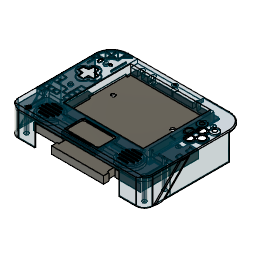
dsCase (Autodesk Fusion 360 design; units mm, degrees)
Autodesk Fusion 360 part; units mm, degrees
(part 1 of 7)
sketch "ds_pcb" plane through (0, 0, 0) normal (0, 0, 1) x (1, 0, 0)
  line L0 (0, 0) -> (0, 63.54)
  line L1 (125.8, 68.8) -> (125.8, 0)
  line L2 (0, 0) -> (0, 63.54)
  line L3 (0, 63.54) -> (24.68, 63.54)
  line L4 (24.68, 63.54) -> (24.68, 68.8)
  line L5 (24.68, 68.8) -> (88.18, 68.8)
  line L6 (24.68, 68.8) -> (88.18, 68.8)
  line L7 (88.18, 68.8) -> (24.68, 68.8)
  line L8 (103.34, 62.2) -> (113.8, 62.2)
  line L9 (125.8, 68.8) -> (115, 68.8)
  line L10 (125.8, 68.8) -> (113.8, 68.8)
  line L11 (113.8, 68.8) -> (113.8, 62.2)
  line L12 (125.8, 68.8) -> (113.8, 68.8)
  line L13 (113.8, 68.8) -> (125.8, 68.8)
  line L14 (88.3, 68.8) -> (88.18, 68.8)
  line L15 (94.8, 68.8) -> (102.3, 68.8)
  line L16 (102.3, 68.8) -> (102.3, 62.2)
  line L17 (102.3, 62.2) -> (103.34, 62.2)
  line L18 (88.3, 68.8) -> (88.3, 63)
  line L19 (94.8, 68.8) -> (94.8, 63)
  line L20 (94.8, 63) -> (88.3, 63)
  line L21 (28.46, 68.8) -> (28.46, 67.3) construction
  line L22 (28.46, 67.3) -> (28.46, 65.3) construction
  circle A0 centre (28.46, 65.3) radius 2
  line L23 (28.46, 65.3) -> (24.68, 65.3) construction
  line L24 (125.8, 68.8) -> (113.8, 68.8)
  line L25 (102.3, 68.8) -> (94.8, 68.8)
  line L26 (98.55, 68.8) -> (98.55, 67.4) construction
  line L27 (98.55, 67.4) -> (98.55, 65.4) construction
  circle A1 centre (98.55, 65.4) radius 2
  line L28 (0, 0) -> (0, 3.5)
  line L29 (0, 3.5) -> (3.5, 3.5) construction
  line L30 (3.5, 3.5) -> (1.5, 3.5) construction
  circle A2 centre (3.5, 3.5) radius 2
  line L31 (125.8, 0) -> (125.8, 3.5)
  line L32 (125.8, 3.5) -> (122.3, 3.5) construction
  line L33 (122.3, 3.5) -> (124.3, 3.5) construction
  circle A3 centre (122.3, 3.5) radius 2
  line L34 (0, 0) -> (34.7, 0)
  line L35 (125.8, 0) -> (96, 0)
  line L36 (37, 10.8) -> (34.7, 10.8)
  line L37 (34.7, 10.8) -> (34.7, 0)
  line L38 (93.7, 10.8) -> (96, 10.8)
  line L39 (96, 10.8) -> (96, 0)
  line L40 (0, 0) -> (34.7, 0)
  line L41 (96, 0) -> (125.8, 0)
  line L42 (72.4833, -13.7) -> (34.7, -13.7)
  line L43 (34.7, -13.7) -> (34.7, -7.2)
  line L44 (72.4833, -13.7) -> (96, -13.7)
  line L45 (96, -13.7) -> (96, -7.2)
  line L46 (96, 10.8) -> (93.7, 10.8)
  line L47 (34.7, 10.8) -> (37, 10.8)
  line L48 (34.7, -13.7) -> (34.7, -7.2)
  line L49 (34.7, -7.2) -> (37, -7.2)
  line L50 (37, -7.2) -> (37, 10.8)
  line L51 (96, -13.7) -> (96, -7.2)
  line L52 (96, -7.2) -> (93.7, -7.2)
  line L53 (93.7, -7.2) -> (93.7, 10.8)
  dimension "d1" = 125.8
  dimension "d3" = 63.54
  dimension "d4" = 101.12
  dimension "d5" = 63.5
  dimension "d11" = 12
  dimension "d14" = 7.5
  dimension "d15" = 31
  dimension "d16" = 6.5
  dimension "d17" = 5.8
  dimension "d20" = 1.5
  dimension "d21" = 2
  dimension "d22" = 4
  dimension "d23" = 1.4
  dimension "d24" = 2
  dimension "d25" = 3.5
  dimension "d26" = 3.5
  dimension "d27" = 2
  dimension "d28" = 3.5
  dimension "d29" = 3.5
  dimension "d30" = 2
  dimension "d31" = 34.7
  dimension "d32" = 29.8
  dimension "d35" = 2.3
  dimension "d36" = 2.3
  dimension "d37" = 6.5
  dimension "d38" = 6.5
  constraint coincident L0.start L2.start
  constraint horizontal L40
  constraint perpendicular L0 L40
  constraint perpendicular L0 L6
  constraint perpendicular L1 L40
  constraint perpendicular L2 L40
  constraint perpendicular L1 L12
  constraint perpendicular L0 L3
  constraint perpendicular L3 L4
  constraint perpendicular L4 L5
  constraint collinear L7 L12
  constraint perpendicular L1 L9
  constraint perpendicular L1 L10
  constraint perpendicular L8 L11
  constraint perpendicular L8 L16
  constraint perpendicular L1 L24
  constraint perpendicular L14 L18
  constraint perpendicular L15 L19
  constraint perpendicular L18 L20
  constraint coincident L7 L21.start
  constraint perpendicular L7 L21
  constraint perpendicular L7 L22
  constraint coincident L22.end A0.centre
  constraint coincident L4 L23.end
  constraint perpendicular L4 L23
  constraint collinear L24 L25
  constraint midpoint L15 L26.start
  constraint perpendicular L15 L26
  constraint parallel L26 L27
  constraint coincident L27.end A1.centre
  constraint coincident L26.end A1
  constraint perpendicular L28 L40
  constraint perpendicular L28 L29
  constraint parallel L29 L30
  constraint coincident L29.end L30.start
  constraint coincident L30.end A2
  constraint perpendicular L31 L40
  constraint perpendicular L31 L32
  constraint parallel L32 L33
  constraint coincident L32.end L33.start
  constraint coincident L33.end A3
  constraint perpendicular L28 L34
  constraint perpendicular L1 L35
  constraint perpendicular L34 L37
  constraint perpendicular L39 L40
  constraint collinear L40 L41
  constraint perpendicular L37 L42
  constraint perpendicular L34 L43
  constraint perpendicular L39 L44
  constraint perpendicular L41 L45
  constraint perpendicular L39 L46
  constraint perpendicular L37 L47
  constraint perpendicular L42 L48
  constraint perpendicular L43 L49
  constraint perpendicular L47 L50
  constraint perpendicular L44 L51
  constraint perpendicular L45 L52
  constraint perpendicular L38 L53
  measures "d1" distance of L0.start L1.end
  measures "d3" distance of L0.start L0.end
  measures "d4" distance of L1.start L4.end
  measures "d5" distance of L4.end L5.end
  measures "d11" distance of L1.start L10.end
  measures "d14" distance of L15.start L15.end
  measures "d15" distance of L1.start L15.start
  measures "d16" distance of L15.start L14.start
  measures "d17" distance of L14.start L18.end
  measures "d20" distance of L21.start L21.end
  measures "d21" distance of L21.end L22.end
  measures "d22" diameter of A0
  measures "d23" distance of L26.start L26.end
  measures "d24" distance of L26.end L27.end
  measures "d25" distance of L0.start L28.end
  measures "d26" distance of L28.end L29.end
  measures "d27" distance of L29.end L30.end
  measures "d28" distance of L1.end L31.end
  measures "d29" distance of L31.end L32.end
  measures "d30" distance of L32.end L33.end
  measures "d31" distance of L0.start L34.end
  measures "d32" distance of L1.end L35.end
  measures "d35" distance of L38.end L38.start
  measures "d36" distance of L36.end L36.start
  measures "d37" distance of L42.end L43.end
  measures "d38" distance of L44.end L45.end
sketch "dsi_screen" plane through (0, 0, 0) normal (0, 0, 1) x (1, 0, 0)
  line L0 (0, 0) -> (0, 79.2)
  line L1 (0, 0) -> (93.9, 0)
  line L2 (0, 79.2) -> (93.9, 79.2)
  line L3 (93.9, 79.2) -> (93.9, 0)
  dimension "d39" = 79.2
  dimension "d40" = 93.9
  constraint coincident L0.start L1.start
  constraint vertical L0
  constraint perpendicular L0 L1
  constraint perpendicular L0 L2
  constraint perpendicular L1 L3
  measures "d39" distance of L0.start L0.end
  measures "d40" distance of L0.start L1.end
sketch "buttons" plane through (0, 0, 0) normal (0, 0, 1) x (1, 0, 0)
  line L0 (0, 0) -> (7.5, 0) construction
  line L1 (3.75, 0) -> (3.75, 3.75) construction
  line L2 (3.75, 0) -> (3.75, -3.75) construction
  line L3 (7.5, 0) -> (11.25, 0) construction
  line L4 (3.75, 3.75) -> (3.75, 7.5) construction
  line L5 (0, 0) -> (-3.75, 0) construction
  line L6 (3.75, -3.75) -> (3.75, -7.5) construction
  circle A0 centre (11.25, 0) radius 3.75
  circle A1 centre (3.75, 7.5) radius 3.75
  circle A2 centre (3.75, -7.5) radius 3.75
  circle A3 centre (-3.75, 0) radius 3.75
  line L7 (15, 0) -> (20, 0) construction
  line L8 (-7.5, 0) -> (-12.5, 0) construction
  line L9 (3.75, 11.25) -> (3.75, 16.25) construction
  line L10 (3.75, -11.25) -> (3.75, -16.25) construction
  line L11 (-12.5, 0) -> (-12.5, -16.25)
  line L12 (-12.5, -16.25) -> (3.75, -16.25)
  line L13 (3.75, -16.25) -> (20, -16.25)
  line L14 (20, -16.25) -> (20, 0)
  line L15 (20, 0) -> (20, 16.25)
  line L16 (20, 16.25) -> (3.75, 16.25)
  line L17 (3.75, 16.25) -> (-12.5, 16.25)
  line L18 (-12.5, 16.25) -> (-12.5, 0)
  line L19 (-12.5, 16.25) -> (-12.5, 26.25)
  line L20 (20, 16.25) -> (20, 26.25)
  line L21 (-12.5, 26.25) -> (20, 26.25)
  dimension "d41" = 7.5
  dimension "d42" = 3.75
  dimension "d43" = 3.75
  dimension "d44" = 3.75
  dimension "d45" = 3.75
  dimension "d46" = 3.75
  dimension "d47" = 3.75
  dimension "d48" = 5
  dimension "d49" = 5
  dimension "d50" = 5
  dimension "d51" = 5
  dimension "d93" = 10
  dimension "d94" = 10
  constraint coincident L0.start L5.start
  constraint horizontal L0
  constraint midpoint L0 L1.start
  constraint perpendicular L0 L1
  constraint perpendicular L0 L2
  constraint perpendicular L1 L3
  constraint parallel L1 L4
  constraint parallel L0 L5
  constraint parallel L2 L6
  constraint coincident L3.end A0.centre
  constraint coincident L0.end A0
  constraint coincident L4.end A1.centre
  constraint coincident L1.end A1
  constraint coincident L6.end A2.centre
  constraint coincident L2.end A2
  constraint coincident L5.end A3.centre
  constraint coincident L0.start A3
  constraint coincident A0 L7.start
  constraint horizontal L7
  constraint coincident A3 L8.start
  constraint parallel L7 L8
  constraint coincident A1 L9.start
  constraint parallel L4 L9
  constraint coincident A2 L10.start
  constraint perpendicular L5 L10
  constraint perpendicular L8 L11
  constraint perpendicular L10 L12
  constraint perpendicular L10 L13
  constraint perpendicular L7 L14
  constraint perpendicular L7 L15
  constraint perpendicular L9 L16
  constraint perpendicular L9 L17
  constraint perpendicular L8 L18
  constraint perpendicular L17 L19
  constraint perpendicular L16 L20
  measures "d41" distance of L0.start L0.end
  measures "d42" distance of L1.start L1.end
  measures "d43" distance of L1.start L2.end
  measures "d44" distance of L0.end L3.end
  measures "d45" distance of L1.end L4.end
  measures "d46" distance of L0.start L5.end
  measures "d47" distance of L2.end L6.end
  measures "d48" distance of L7.start L7.end
  measures "d49" distance of L8.start L8.end
  measures "d50" distance of L9.start L9.end
  measures "d51" distance of L10.start L10.end
  measures "d93" distance of L17.end L19.end
  measures "d94" distance of L15.end L20.end
sketch "cross" plane through (0, 0, 0) normal (0, 0, 1) x (1, 0, 0)
  line L0 (9.25, -9.25) -> (9.25, -16.25) construction
  line L1 (18.5, 0) -> (25.5, 0) construction
  line L2 (0, 0) -> (-7, 0) construction
  line L3 (0, 0) -> (0, 3.25)
  line L4 (0, 3.25) -> (0, -3.25)
  line L5 (18.5, 0) -> (18.5, 3.25)
  line L6 (18.5, 0) -> (18.5, -3.25)
  line L7 (9.25, 9.25) -> (12.5, 9.25)
  line L8 (9.25, 9.25) -> (6, 9.25)
  line L9 (9.25, -9.25) -> (12.5, -9.25)
  line L10 (9.25, -9.25) -> (6, -9.25)
  line L11 (9.25, 9.25) -> (9.25, 16.25) construction
  line L12 (0, 3.25) -> (6, 3.25)
  line L13 (12.5, 3.25) -> (18.5, 3.25)
  line L14 (6, 9.25) -> (6, 3.25)
  line L15 (6, -3.25) -> (6, -9.25)
  line L16 (12.5, 9.25) -> (12.5, 3.25)
  line L17 (12.5, -3.25) -> (12.5, -9.25)
  line L18 (0, -3.25) -> (6, -3.25)
  line L19 (12.5, -3.25) -> (18.5, -3.25)
  line L20 (9.25, 16.25) -> (-7, 16.25)
  line L21 (-7, 16.25) -> (-7, 0)
  line L22 (-7, 0) -> (-7, -16.25)
  line L23 (-7, -16.25) -> (9.25, -16.25)
  line L24 (9.25, -16.25) -> (25.5, -16.25)
  line L25 (25.5, -16.25) -> (25.5, 0)
  line L26 (25.5, 0) -> (25.5, 16.25)
  line L27 (25.5, 16.25) -> (9.25, 16.25)
  dimension "d52" = 18.5
  dimension "d59" = 3.25
  dimension "d60" = 6.5
  dimension "d61" = 3.25
  dimension "d62" = 3.25
  dimension "d63" = 3.25
  dimension "d64" = 3.25
  dimension "d65" = 3.25
  dimension "d66" = 3.25
  constraint coincident L2.start L3.start
  constraint perpendicular L2 L3
  constraint parallel L3 L4
  constraint perpendicular L0 L9
  constraint collinear L12 L13
  constraint collinear L14 L15
  constraint coincident L3 L2.start
  constraint collinear L16 L17
  constraint coincident L17.start L18
  constraint collinear L18 L19
  constraint perpendicular L11 L20
  constraint perpendicular L2 L21
  constraint perpendicular L2 L22
  constraint perpendicular L0 L23
  constraint perpendicular L0 L24
  constraint perpendicular L1 L25
  constraint perpendicular L20 L26
  constraint perpendicular L11 L27
  measures "d52" distance of L2.start L1.start
  measures "d59" distance of L2.start L3.end
  measures "d60" distance of L3.end L4.end
  measures "d61" distance of L1.start L5.end
  measures "d62" distance of L1.start L6.end
  measures "d63" distance of L7.start L7.end
  measures "d64" distance of L7.start L8.end
  measures "d65" distance of L0.start L9.end
  measures "d66" distance of L0.start L10.end
extrude "Extrude1" add sketch "dsi_screen" along normal blind 5.6 makes body 1
extrude "Extrude2" add sketch "ds_pcb" against normal blind 0.7 separate body makes body 2
move_body "Move1" bodies 1 to x (1, 0, 0) y (0, 1, 0) z (0, 0, 1) at (0, 0, 10)
extrude "Extrude3" add sketch "cross" along normal blind 2.5 separate body makes body 3
move_body "Move2" bodies 3 to x (1, 0, 0) y (0, 1, 0) z (0, 0, 1) at (-30, 60, 12)
sketch "Sketch5" plane through (0, 0, 15.6) normal (0, 0, 1) x (-1, 0, 0)
  line L0 (0, 0) -> (-93.9, 0)
  line L1 (-93.9, 0) -> (-93.9, -79.2)
  line L2 (-93.9, -79.2) -> (0, -79.2)
  line L3 (0, -79.2) -> (0, 0)
  line L4 (0, -79.2) -> (0, -57.7) construction
  line L5 (0, -57.7) -> (-93.9, -57.7) construction
  dimension "d75" = 21.5
  constraint coincident L2.end L3.start
  constraint perpendicular L2 L4
  constraint coincident L1 L5.end
  constraint perpendicular L1 L5
  measures "d75" distance of L2.end L4.end
move_body "Move4" bodies 3 to x (1, 0, 0) y (0, 1, 0) z (0, 0, 1) at (-2, 0, 0)
move_body "Move5" bodies 3 to x (1, 0, 0) y (0, 1, 0) z (0, 0, 1) at (6.5, -18.55, 1.1)
extrude "Extrude5" add sketch "buttons" along normal blind 2.5 separate body makes body 4
move_body "Move7" bodies 4 to x (1, 0, 0) y (0, 1, 0) z (0, 0, 1) at (106.4, 31.45, 13.1)
move_body "Move8" bodies 1 to x (1, 0, 0) y (0, 1, 0) z (0, 0, 1) at (0, -4.1, 0)
move_body "Move9" bodies 4 to x (1, 0, 0) y (0, 1, 0) z (0, 0, 1) at (0, 10, 0)
sketch "Sketch14" plane through (0, 0, 15.6) normal (0, 0, 1) x (-1, 0, 0)
  circle A0 centre (-102.65, -41.45) radius 3.75
  circle A1 centre (-110.15, -33.95) radius 3.75
  circle A2 centre (-117.65, -41.45) radius 3.75
  circle A3 centre (-110.15, -48.95) radius 3.75
  line L0 (-93.9, -67.7) -> (-93.9, -25.2)
  line L1 (-93.9, -25.2) -> (-126.4, -25.2)
  line L2 (-126.4, -25.2) -> (-126.4, -67.7)
  line L3 (-126.4, -67.7) -> (-93.9, -67.7)
  line L4 (-110.15, -48.95) -> (-117.65, -41.45) construction
  line L5 (-117.65, -41.45) -> (-110.15, -41.45) construction
  line L6 (-110.15, -41.45) -> (-110.15, -48.95) construction
  line L7 (-110.15, -48.95) -> (-102.6547, -56.4453) construction
  line L8 (-110.15, -48.95) -> (-117.6453, -56.4453) construction
  circle A4 centre (-102.6547, -56.4453) radius 2.35
  circle A5 centre (-117.6453, -56.4453) radius 2.35
  dimension "d96" = 10.6
  dimension "d97" = 10.6
  dimension "d98" = 4.7
  dimension "d99" = 4.7
  constraint coincident A3.centre L4.start
  constraint coincident A2.centre L4.end
  constraint horizontal L5
  constraint perpendicular L5 L6
  constraint parallel L4 L7
  constraint perpendicular L4 L8
  constraint coincident L7.end A4.centre
  constraint coincident L8.end A5.centre
  measures "d96" distance of A3.centre L7.end
  measures "d97" distance of A3.centre L8.end
  measures "d98" diameter of A4
  measures "d99" diameter of A5
extrude "Extrude7" cut sketch "Sketch14" against normal blind 3 contours A4 | A5 bodies 4
sketch "Sketch15" plane through (0, 0, 15.6) normal (0, 0, 1) x (-1, 0, 0)
  line L0 (0, 4.1) -> (-93.9, 4.1)
  line L1 (-93.9, 4.1) -> (-93.9, -75.1)
  line L2 (-93.9, -75.1) -> (0, -75.1)
  line L3 (0, -75.1) -> (0, 4.1)
  line L4 (-46.95, -75.1) -> (-46.95, -85.1)
  line L5 (-46.95, -85.1) -> (32.5, -85.1)
  line L6 (32.5, -85.1) -> (32.5, -57.7)
  line L7 (32.5, -57.7) -> (0, -57.7)
  line L8 (0, -75.1) -> (0, -57.7)
  line L9 (0, -75.1) -> (-93.9, -75.1)
  line L10 (-93.9, -75.1) -> (-93.9, -67.7)
  line L11 (-93.9, -67.7) -> (-126.4, -67.7)
  line L12 (-126.4, -67.7) -> (-126.4, -85.1)
  line L13 (-126.4, -85.1) -> (-46.95, -85.1)
  point P0 (32.5, -57.7)
  point P1 (0, -57.7)
  point P2 (0, -57.7)
  point P3 (-93.9, -67.7)
  point P4 (-93.9, -67.7)
  point P5 (-126.4, -67.7)
  dimension "d102" = 10
  constraint midpoint L2 L4.start
  constraint perpendicular L2 L4
  constraint perpendicular L4 L5
  constraint coincident P0 L6.end
  constraint perpendicular L5 L6
  constraint coincident P2 P1
  constraint coincident L2.end L3.start
  constraint coincident L1.end L2.start
  constraint coincident P4 P3
  constraint coincident P5 L11.end
  constraint perpendicular L5 L12
  constraint perpendicular L4 L13
  measures "d102" distance of L4.start L4.end
extrude "Extrude8" add sketch "Sketch15" against normal blind 2.5 separate body contours L2 L3 L4 L5 L6 L7 L8 L9 | L1 L2 L4 L9 L10 L11 L12 L13 makes body 5
sketch "Sketch16" plane through (0, 0, 15.6) normal (0, 0, 1) x (-1, 0, 0)
  line L0 (0, -75.1) -> (-93.9, -75.1)
  line L1 (-93.9, -75.1) -> (-93.9, -67.7)
  line L2 (-93.9, -67.7) -> (-126.4, -67.7)
  line L3 (-126.4, -67.7) -> (-126.4, -85.1)
  line L4 (-126.4, -85.1) -> (32.5, -85.1)
  line L5 (32.5, -85.1) -> (32.5, -57.7)
  line L6 (32.5, -57.7) -> (0, -57.7)
  line L7 (0, -57.7) -> (0, -75.1)
  line L8 (-126.4, -85.1) -> (-106.4, -85.1)
  line L9 (-106.4, -85.1) -> (-106.4, -65.1)
  line L10 (-126.4, -85.1) -> (-126.4, -65.1)
  arc A0 (-126.4, -65.1) -> (-106.4, -85.1) centre (-106.4, -65.1) ccw
  line L11 (-46.95, -75.1) -> (-46.95, -92.0234) construction
  arc A1 (12.5, -85.1) -> (32.5, -65.1) centre (12.5, -65.1) ccw
  line L12 (32.5, -85.1) -> (32.5, -65.1)
  line L13 (32.5, -85.1) -> (12.5, -85.1)
  dimension "d105" = 20
  dimension "d106" = 20
  constraint coincident L3.end L4.start
  constraint perpendicular L3 L8
  constraint perpendicular L2 L9
  constraint coincident L9.end A0.centre
  constraint tangent L10 A0
  constraint midpoint L0 L11.start
  constraint perpendicular L4 L11
  constraint symmetric L3.end L11 L4.end
  constraint symmetric L8.end L11 A1.start
  constraint symmetric L10.end L11 A1.end
  constraint symmetric A0 L11 A1
  measures "d105" distance of L3.end L8.end
  measures "d106" distance of L8.end L9.end
extrude "Extrude9" cut sketch "Sketch16" against normal blind 2.5 contours L4 L5 A1 L12 L13 | L2 L3 L4 L8 L10 A0 | L2 L10 A0 bodies 4 5
sketch "Controls" plane through (0, 0, 15.6) normal (0, 0, 1) x (-1, 0, 0)
  line L0 (0, 4.1) -> (-93.9, 4.1)
  line L1 (-93.9, 4.1) -> (-93.9, -75.1)
  line L2 (-93.9, -75.1) -> (0, -75.1)
  line L3 (0, -75.1) -> (0, 4.1)
  line L4 (-93.9, 4.1) -> (0, 4.1)
  line L5 (0, 4.1) -> (0, -75.1)
  line L6 (0, -75.1) -> (-93.9, -75.1)
  line L7 (-93.9, -75.1) -> (-93.9, 4.1)
  line L8 (0, -25.2) -> (32.5, -25.2)
  line L9 (32.5, -25.2) -> (32.5, -65.1)
  arc A0 (12.5, -85.1) -> (32.5, -65.1) centre (12.5, -65.1) ccw
  line L10 (12.5, -85.1) -> (-106.4, -85.1)
  line L11 (-93.9, -25.2) -> (-126.4, -25.2)
  line L12 (-126.4, -25.2) -> (-93.9, -25.2)
  arc A1 (12.5, -85.1) -> (32.5, -65.1) centre (12.5, -65.1) ccw
  line L13 (-126.4, -25.2) -> (-126.4, -65.1)
  arc A2 (-126.4, -65.1) -> (-106.4, -85.1) centre (-106.4, -65.1) ccw
  line L14 (19.5, -44.7) -> (19.5, -50.7)
  line L15 (19.5, -50.7) -> (19.5, -44.7)
  line L16 (19.5, -44.7) -> (25.5, -44.7)
  line L17 (25.5, -44.7) -> (25.5, -38.2)
  line L18 (25.5, -38.2) -> (19.5, -38.2)
  line L19 (19.5, -38.2) -> (19.5, -32.2)
  line L20 (19.5, -32.2) -> (13, -32.2)
  line L21 (13, -32.2) -> (13, -38.2)
  line L22 (13, -38.2) -> (7, -38.2)
  line L23 (7, -38.2) -> (7, -44.7)
  line L24 (7, -44.7) -> (13, -44.7)
  line L25 (13, -44.7) -> (13, -50.7)
  line L26 (13, -50.7) -> (19.5, -50.7)
  circle A3 centre (-117.65, -41.45) radius 3.75
  circle A4 centre (-110.15, -48.95) radius 3.75
  circle A5 centre (-110.15, -33.95) radius 3.75
  circle A6 centre (-117.65, -41.45) radius 3.75
  circle A7 centre (-110.15, -48.95) radius 3.75
  circle A8 centre (-110.15, -33.95) radius 3.75
  circle A9 centre (-102.65, -41.45) radius 3.75
  circle A10 centre (-102.6547, -56.4453) radius 2.35
  circle A11 centre (-102.6547, -56.4453) radius 2.35
  circle A12 centre (-117.6453, -56.4453) radius 2.35
  circle A13 centre (-102.6547, -56.4453) radius 2.35
  circle A14 centre (-117.6453, -56.4453) radius 2.35
  line L27 (-110.15, -33.95) -> (-110.15, -40) construction
  line L28 (-110.15, -33.95) -> (-110.15, -37.7) construction
  line L29 (-110.15, -37.7) -> (-110.15, 35.3) construction
  line L30 (-126.4, -25.2) -> (-126.4, 25.3)
  line L31 (32.5, -25.2) -> (32.5, 25.3)
  line L32 (-110.15, 35.3) -> (-116.4, 35.3)
  line L33 (-110.15, 35.3) -> (22.5, 35.3)
  line L34 (0, 4.1) -> (0, 35.3) construction
  circle A15 centre (0, 19.7) radius 11.5
  line L35 (-93.9, 4.1) -> (-93.9, 35.3) construction
  circle A16 centre (-93.9, 19.7) radius 11.5
  line L36 (-116.4, 35.3) -> (-116.4, 25.3) construction
  arc A17 (-116.4, 35.3) -> (-126.4, 25.3) centre (-116.4, 25.3) ccw
  line L37 (22.5, 35.3) -> (22.5, 25.3) construction
  arc A18 (32.5, 25.3) -> (22.5, 35.3) centre (22.5, 25.3) ccw
  point P0 (0, -25.2)
  point P1 (32.5, -25.2)
  point P2 (-126.2303, -67.7)
  point P3 (-126.4, -25.2)
  point P4 (-126.4, -25.2)
  point P5 (-93.9, -25.2)
  point P6 (19.5, -50.7)
  point P7 (19.5, -44.7)
  point P8 (19.5, -44.7)
  point P9 (25.5, -44.7)
  point P10 (25.5, -38.2)
  point P11 (19.5, -38.2)
  point P12 (19.5, -32.2)
  point P13 (13, -32.2)
  point P14 (13, -38.2)
  point P15 (7, -38.2)
  point P16 (7, -44.7)
  point P17 (13, -44.7)
  point P18 (13, -50.7)
  point P19 (-98.9, -41.45)
  point P20 (-119.9953, -56.4453)
  dimension "d127" = 73
  dimension "d128" = 23
  dimension "d129" = 23
  dimension "d131" = 10
  dimension "d133" = 10
  constraint coincident L0.end L1.start
  constraint coincident L0.start L3.end
  constraint coincident L2.end L3.start
  constraint coincident L1.end L2.start
  constraint coincident P0 L8.start
  constraint coincident P1 L8.end
  constraint coincident L9.end A0.end
  constraint coincident A0.start L10.start
  constraint coincident L10.end A2.end
  constraint coincident P4 P3
  constraint coincident P5 L11.start
  constraint concentric A0 A1
  constraint coincident L13.end A2.start
  constraint coincident L13.end A2
  constraint coincident P6 L14.end
  constraint coincident P8 P7
  constraint coincident P9 L16.end
  constraint coincident P10 L17.end
  constraint coincident P11 L18.end
  constraint coincident P12 L19.end
  constraint coincident P13 L20.end
  constraint coincident P14 L21.end
  constraint coincident P15 L22.end
  constraint coincident P16 L23.end
  constraint coincident P17 L24.end
  constraint coincident P18 L25.end
  constraint concentric A3 A6
  constraint concentric A4 A7
  constraint concentric A5 A8
  constraint coincident P19 A9
  constraint concentric A11 A13
  constraint concentric A12 A14
  constraint coincident A5.centre A8.centre
  constraint perpendicular L12 L27
  constraint coincident L27 L28.end
  constraint coincident A8 L28.end
  constraint perpendicular L11 L29
  constraint perpendicular L12 L30
  constraint perpendicular L30 L32
  constraint perpendicular L31 L33
  constraint coincident L33 L34.end
  constraint perpendicular L33 L34
  constraint midpoint L34 A15.centre
  constraint coincident L33 L35.end
  constraint perpendicular L33 L35
  constraint midpoint L35 A16.centre
  constraint coincident L36.end A17.centre
  constraint coincident L37.end A18.centre
  measures "d127" distance of L28.end L29.end
  measures "d128" diameter of A15
  measures "d129" diameter of A16
  measures "d131" distance of L32.end L36.end
  measures "d133" distance of L33.end L37.end
sketch "Sketch19" plane through (0, 0, 0) normal (0, 0, 1) x (1, 0, 0)
  line L0 (0, -35) -> (37.5, -35)
  line L1 (37.5, -35) -> (37.5, -54.4)
  line L2 (37.5, -54.4) -> (0, -54.4)
  line L3 (0, -54.4) -> (0, -35)
  dimension "d109" = 37.5
  dimension "d110" = 19.4
  constraint horizontal L0
  constraint perpendicular L0 L1
  constraint perpendicular L1 L2
  constraint perpendicular L2 L3
  measures "d109" distance of L0.start L0.end
  measures "d110" distance of L0.end L1.end
extrude "Extrude10" add sketch "Sketch19" along normal blind 2 separate body makes body 6
fillet "Fillet1" radius 3 4 edges at (37.5, -35, 1) (37.5, -54.4, 1) (0, -54.4, 1) (0, -35, 1) on bodies 6
move_body "Move10" bodies 6 to x (1, 0, 0) y (0, 1, 0) z (0, 0, 1) at (30, 30, 0)
move_body "Move11" bodies 6 to x (1, 0, 0) y (0, 1, 0) z (0, 0, 1) at (-1.8, 0, 0)
move_body "Move12" bodies 6 to x (1, 0, 0) y (0, 1, 0) z (0, 0, 1) at (0, -5, 0)
move_body "Move13" bodies 6 to x (1, 0, 0) y (0, 1, 0) z (0, 0, 1) at (0, 0, 13.5)
move_body "Move14" bodies 6 to x (1, 0, 0) y (0, 1, 0) z (0, 0, 1) at (0, 0, -7)
sketch "Sketch20" plane through (0, 0, 6.5) normal (0, 0, -1) x (1, 0, 0)
  arc A0 (28.2, 13) -> (31.2, 10) centre (31.2, 13) ccw
  line L0 (31.2, 10) -> (62.7, 10)
  arc A1 (62.7, 10) -> (65.7, 13) centre (62.7, 13) ccw
  line L1 (65.7, 13) -> (65.7, 26.4)
  arc A2 (65.7, 26.4) -> (62.7, 29.4) centre (62.7, 26.4) ccw
  line L2 (62.7, 29.4) -> (31.2, 29.4)
  arc A3 (31.2, 29.4) -> (28.2, 26.4) centre (31.2, 26.4) ccw
  line L3 (28.2, 26.4) -> (28.2, 13)
  line L4 (46.95, 10) -> (46.95, 5)
  line L5 (46.95, 29.4) -> (46.95, 34.4)
  line L6 (28.2, 19.7) -> (27.2, 19.7)
  line L7 (65.7, 19.7) -> (66.7, 19.7)
  line L8 (46.95, 5) -> (27.2, 5)
  line L9 (46.95, 34.4) -> (66.7, 34.4)
  line L10 (27.2, 5) -> (66.7, 5)
  line L11 (66.7, 5) -> (66.7, 34.4)
  line L12 (66.7, 34.4) -> (27.2, 34.4)
  line L13 (27.2, 34.4) -> (27.2, 5)
  dimension "d115" = 5
  dimension "d116" = 5
  dimension "d117" = 1
  dimension "d118" = 1
  constraint midpoint L0 L4.start
  constraint perpendicular L0 L4
  constraint midpoint L2 L5.start
  constraint perpendicular L2 L5
  constraint midpoint L3 L6.start
  constraint perpendicular L3 L6
  constraint midpoint L1 L7.start
  constraint perpendicular L1 L7
  constraint perpendicular L4 L8
  constraint perpendicular L5 L9
  constraint horizontal L10
  constraint vertical L11
  constraint horizontal L12
  constraint vertical L13
  measures "d115" distance of L4.start L4.end
  measures "d116" distance of L5.start L5.end
  measures "d117" distance of L6.start L6.end
  measures "d118" distance of L7.start L7.end
extrude "Extrude11" add sketch "Sketch20" along normal blind 1.6 bodies 6
move_body "Move15" bodies 6 to x (1, 0, 0) y (0, 1, 0) z (0, 0, 1) at (0, 0.5, 7)
move_body "Move16" bodies 2 to x (1, 0, 0) y (0, 1, 0) z (0, 0, 1) at (0, -21, 0)
move_body "Move17" bodies 2 to x (1, 0, 0) y (0, 1, 0) z (0, 0, 1) at (-15, 0, 0)
move_body "Move18" bodies 2 to x (1, 0, 0) y (0, 1, 0) z (0, 0, 1) at (-3, 0, 0)
move_body "Move19" bodies 2 to x (1, 0, 0) y (0, 1, 0) z (0, 0, 1) at (-0.4, 0, 0)
sketch "Sketch21" plane through (0, 0, 13.1) normal (0, 0, -1) x (1, 0, 0)
  line L0 (-19.5, -32.2) -> (-13, -32.2)
  line L1 (-13, -32.2) -> (-13, -38.2)
  line L2 (-13, -38.2) -> (-7, -38.2)
  line L3 (-7, -38.2) -> (-7, -44.7)
  line L4 (-7, -44.7) -> (-13, -44.7)
  line L5 (-13, -44.7) -> (-13, -50.7)
  line L6 (-13, -50.7) -> (-19.5, -50.7)
  line L7 (-19.5, -50.7) -> (-19.5, -44.7)
  line L8 (-19.5, -44.7) -> (-25.5, -44.7)
  line L9 (-25.5, -44.7) -> (-25.5, -38.2)
  line L10 (-25.5, -38.2) -> (-19.5, -38.2)
  line L11 (-19.5, -38.2) -> (-19.5, -32.2)
  line L12 (-32.5, -57.7) -> (0, -57.7)
  line L13 (0, -57.7) -> (0, -25.2)
  line L14 (0, -25.2) -> (-32.5, -25.2)
  line L15 (-32.5, -25.2) -> (-32.5, -57.7)
  line L16 (0, -57.7) -> (-32.5, -57.7)
  line L17 (-32.5, -57.7) -> (-32.5, -25.2)
  line L18 (-32.5, -25.2) -> (0, -25.2)
  line L19 (0, -25.2) -> (0, -57.7)
  line L20 (-13, -50.7) -> (-19.5, -50.7)
  line L21 (-19.5, -50.7) -> (-19.5, -44.7)
  line L22 (-19.5, -44.7) -> (-25.5, -44.7)
  line L23 (-25.5, -44.7) -> (-25.5, -38.2)
  line L24 (-25.5, -38.2) -> (-19.5, -38.2)
  line L25 (-19.5, -38.2) -> (-19.5, -32.2)
  line L26 (-19.5, -32.2) -> (-13, -32.2)
  line L27 (-13, -32.2) -> (-13, -38.2)
  line L28 (-13, -38.2) -> (-7, -38.2)
  line L29 (-7, -38.2) -> (-7, -44.7)
  line L30 (-7, -44.7) -> (-13, -44.7)
  line L31 (-13, -44.7) -> (-13, -50.7)
  line L32 (-13, -50.7) -> (-13, -44.7)
  constraint coincident L12.end L13.start
  constraint coincident L12.start L15.end
  constraint coincident L14.end L15.start
  constraint coincident L13.end L14.start
  constraint coincident L5.end L6.start
  constraint coincident L6.end L7.start
  constraint coincident L7.end L8.start
  constraint coincident L8.end L9.start
  constraint coincident L9.end L10.start
  constraint coincident L10.end L11.start
  constraint coincident L0.start L11.end
  constraint coincident L0.end L1.start
  constraint coincident L1.end L2.start
  constraint coincident L2.end L3.start
  constraint coincident L3.end L4.start
  constraint coincident L4.end L5.start
extrude "Extrude12" cut sketch "Sketch21" against normal blind 1.5 bodies 3
sketch "Sketch22" plane through (0, 0, 14.6) normal (0, 0, -1) x (1, 0, 0)
  line L0 (-13, -50.7) -> (-19.5, -50.7)
  line L1 (-19.5, -50.7) -> (-19.5, -44.7)
  line L2 (-19.5, -44.7) -> (-25.5, -44.7)
  line L3 (-25.5, -44.7) -> (-25.5, -38.2)
  line L4 (-25.5, -38.2) -> (-19.5, -38.2)
  line L5 (-19.5, -38.2) -> (-19.5, -32.2)
  line L6 (-19.5, -32.2) -> (-13, -32.2)
  line L7 (-13, -32.2) -> (-13, -38.2)
  line L8 (-13, -38.2) -> (-7, -38.2)
  line L9 (-7, -38.2) -> (-7, -44.7)
  line L10 (-7, -44.7) -> (-13, -44.7)
  line L11 (-13, -44.7) -> (-13, -50.7)
  line L12 (0, -25.2) -> (-32.5, -25.2)
  line L13 (-32.5, -25.2) -> (-32.5, -57.7)
  line L14 (-32.5, -57.7) -> (0, -57.7)
  line L15 (0, -57.7) -> (0, -25.2)
  line L16 (-19.5, -44.7) -> (-19.5, -47)
  line L17 (-19.5, -44.7) -> (-21.8, -44.7)
  arc A0 (-21.8, -44.7) -> (-19.5, -47) centre (-19.5, -44.7) ccw construction
  line L18 (-16.25, -50.7) -> (-16.25, -32.2) construction
  line L19 (-7, -41.45) -> (-25.5, -41.45) construction
  line L20 (-21.1263, -46.3263) -> (-19.5, -44.7) construction
  circle A1 centre (-16.25, -41.45) radius 6.8962
  dimension "d136" = 4.6
  constraint coincident L1.end L2.start
  constraint coincident L1 L16.end
  constraint coincident L2 L17.end
  constraint midpoint L0 L18.start
  constraint midpoint L6 L18.end
  constraint midpoint L9 L19.start
  constraint midpoint L3 L19.end
  constraint midpoint A0 L20.start
  constraint midpoint L19 A1.centre
  constraint coincident L20.start A1
  measures "d136" diameter of A0
extrude "Extrude13" cut sketch "Sketch22" against normal blind 0.5 contours L10 L11 A1 | L1 L2 L16 L17 A1 | L4 L5 A1 | L7 L8 A1 bodies 3
sketch "Sketch23" plane through (0, 0, 14.6) normal (0, 0, -1) x (1, 0, 0)
  arc A0 (-13, -47.5324) -> (-10.1676, -44.7) centre (-16.25, -41.45) ccw
  line L0 (-13, -47.5324) -> (-13, -50.7)
  line L1 (-13, -50.7) -> (-19.5, -50.7)
  line L2 (-19.5, -50.7) -> (-19.5, -47.5324)
  arc A1 (-22.3324, -44.7) -> (-19.5, -47.5324) centre (-16.25, -41.45) ccw
  line L3 (-22.3324, -44.7) -> (-25.5, -44.7)
  line L4 (-25.5, -44.7) -> (-25.5, -38.2)
  line L5 (-25.5, -38.2) -> (-22.3324, -38.2)
  arc A2 (-19.5, -35.3676) -> (-22.3324, -38.2) centre (-16.25, -41.45) ccw
  line L6 (-19.5, -35.3676) -> (-19.5, -32.2)
  line L7 (-19.5, -32.2) -> (-13, -32.2)
  line L8 (-13, -32.2) -> (-13, -35.3676)
  arc A3 (-10.1676, -38.2) -> (-13, -35.3676) centre (-16.25, -41.45) ccw
  line L9 (-10.1676, -38.2) -> (-7, -38.2)
  line L10 (-7, -38.2) -> (-7, -44.7)
  line L11 (-7, -44.7) -> (-10.1676, -44.7)
  line L12 (0, -25.2) -> (-32.5, -25.2)
  line L13 (-32.5, -25.2) -> (-32.5, -57.7)
  line L14 (-32.5, -57.7) -> (0, -57.7)
  line L15 (0, -57.7) -> (0, -25.2)
  line L16 (-7, -41.45) -> (-3.75, -41.45)
  line L17 (-25.5, -41.45) -> (-28.75, -41.45)
  line L18 (-16.25, -50.7) -> (-16.25, -53.95)
  line L19 (-16.25, -32.2) -> (-16.25, -28.95)
  line L20 (-10.1676, -41.45) -> (-7, -41.45)
  line L21 (-19.5, -50.7) -> (-19.5, -44.7)
  line L22 (-19.5, -47.7) -> (-16.25, -47.7)
  line L23 (-19.5, -38.2) -> (-25.5, -38.2)
  line L24 (-22.5, -38.2) -> (-22.5, -41.45)
  line L25 (-19.5, -32.2) -> (-19.5, -38.2)
  line L26 (-19.5, -35.2) -> (-16.25, -35.2)
  arc A4 (-9.5307, -48.3426) -> (-9.5307, -34.5574) centre (-10.1676, -41.45) ccw
  arc A5 (-22.5, -47.7) -> (-10.0022, -47.8655) centre (-16.25, -47.7) ccw
  arc A6 (-22.9827, -48.1827) -> (-9.5307, -48.3426) centre (-16.25, -47.7) ccw
  arc A7 (-19.5346, -47.5137) -> (-19.5, -47.4967) centre (-22.5, -41.45) ccw
  arc A8 (-22.5, -35.2) -> (-22.5, -47.7) centre (-22.5, -41.45) ccw
  arc A9 (-22.9827, -34.7173) -> (-22.9827, -48.1827) centre (-22.5, -41.45) ccw
  arc A10 (-10.1863, -38.1654) -> (-10.1676, -38.127) centre (-16.25, -35.2) ccw
  arc A11 (-9.5307, -34.5574) -> (-22.9827, -34.7173) centre (-16.25, -35.2) ccw
  arc A12 (-10.0022, -35.0345) -> (-22.5, -35.2) centre (-16.25, -35.2) ccw
  line L27 (-10.1676, -38.127) -> (-10.1676, -41.45)
  line L28 (-10.1676, -38.2) -> (-10.1676, -38.127)
  arc A13 (-10.0022, -47.8655) -> (-10.0022, -35.0345) centre (-10.1676, -41.45) ccw
  dimension "d139" = 3.25
  dimension "d140" = 3.25
  dimension "d141" = 3.25
  dimension "d142" = 3.25
  dimension "d146" = 13.5
  dimension "d147" = 13.844
  constraint midpoint L10 L16.start
  constraint perpendicular L10 L16
  constraint midpoint L4 L17.start
  constraint perpendicular L4 L17
  constraint midpoint L1 L18.start
  constraint perpendicular L1 L18
  constraint midpoint L7 L19.start
  constraint perpendicular L7 L19
  constraint coincident A3.start L9.start
  constraint perpendicular L9 L28
  constraint perpendicular L10 L20
  constraint coincident L20.start A4.centre
  constraint coincident L16.end A13
  constraint midpoint L21 L22.start
  constraint perpendicular L18 L22
  constraint midpoint L23 L24.start
  constraint perpendicular L17 L24
  constraint midpoint L25 L26.start
  constraint perpendicular L19 L26
  constraint coincident A3 A10.start
  constraint coincident L21 A7.end
  constraint coincident A1 A7.start
  constraint concentric A10 A11
  measures "d139" distance of L16.start L16.end
  measures "d140" distance of L17.start L17.end
  measures "d141" distance of L18.start L18.end
  measures "d142" distance of L19.start L19.end
  measures "d146" diameter of A10
  measures "d147" diameter of A4
extrude "Extrude14" add sketch "Sketch23" along normal blind 0.8 contours A4 A6 A9 A11 bodies 3
extrude "Extrude15" cut 1 faces at (107.8812, 64.6776, 13.1) along direction (0, 0, 1) blind 1.5 on bodies 4 bodies 4
sketch "Sketch24" plane through (0, 0, 14.6) normal (0, 0, -1) x (1, 0, 0)
  arc A0 (126.2303, -67.7) -> (126.4, -65.1) centre (106.4, -65.1) ccw
  line L0 (126.4, -65.1) -> (126.4, -25.2)
  line L1 (126.4, -25.2) -> (93.9, -25.2)
  line L2 (93.9, -25.2) -> (93.9, -67.7)
  line L3 (93.9, -67.7) -> (126.2303, -67.7)
  circle A1 centre (110.15, -48.95) radius 3.75
  circle A2 centre (117.65, -41.45) radius 3.75
  circle A3 centre (110.15, -33.95) radius 3.75
  circle A4 centre (102.65, -41.45) radius 3.75
  circle A5 centre (117.6453, -56.4453) radius 2.35
  circle A6 centre (102.6547, -56.4453) radius 2.35
  circle A7 centre (110.15, -33.95) radius 3.85
  circle A8 centre (102.65, -41.45) radius 3.85
  circle A9 centre (110.15, -48.95) radius 3.85
  circle A10 centre (117.65, -41.45) radius 3.85
  dimension "d152" = 7.7
  dimension "d153" = 7.7
  dimension "d154" = 7.7
  dimension "d155" = 7.7
  constraint concentric A3 A7
  constraint concentric A4 A8
  constraint concentric A1 A9
  constraint concentric A2 A10
  measures "d152" diameter of A7
  measures "d153" diameter of A8
  measures "d154" diameter of A9
  measures "d155" diameter of A10
extrude "Extrude16" cut sketch "Sketch24" against normal blind 1 contours A7 | A8 | A9 | A10 bodies 4
sketch "Sketch25" plane through (0, 0, 14.6) normal (0, 0, -1) x (1, 0, 0)
  circle A0 centre (110.15, -48.95) radius 3.85
  circle A1 centre (117.65, -41.45) radius 3.85
  circle A2 centre (102.65, -41.45) radius 3.85
  circle A3 centre (110.15, -33.95) radius 3.85
  arc A4 (126.2303, -67.7) -> (126.4, -65.1) centre (106.4, -65.1) ccw
  line L0 (126.4, -65.1) -> (126.4, -25.2)
  line L1 (126.4, -25.2) -> (93.9, -25.2)
  line L2 (93.9, -25.2) -> (93.9, -67.7)
  line L3 (93.9, -67.7) -> (126.2303, -67.7)
  circle A5 centre (117.6453, -56.4453) radius 2.35
  circle A6 centre (102.6547, -56.4453) radius 2.35
  circle A7 centre (110.15, -48.95) radius 5.05
  circle A8 centre (117.65, -41.45) radius 5.05
  circle A9 centre (102.65, -41.45) radius 5.05
  circle A10 centre (110.15, -33.95) radius 5.05
  dimension "d158" = 10.1
  dimension "d159" = 10.1
  dimension "d160" = 10.1
  dimension "d161" = 10.1
  constraint concentric A0 A7
  constraint concentric A1 A8
  constraint concentric A2 A9
  constraint concentric A3 A10
  measures "d158" diameter of A7
  measures "d159" diameter of A8
  measures "d160" diameter of A9
  measures "d161" diameter of A10
extrude "Extrude18" cut sketch "Sketch25" against normal blind 0.5 contours A7 | A8 | A9 | A10 bodies 4
sketch "Sketch27" plane through (0, 0, 14.6) normal (0, 0, -1) x (1, 0, 0)
  line L0 (110.15, -48.95) -> (117.65, -41.45) construction
  line L1 (117.65, -41.45) -> (110.15, -33.95) construction
  line L2 (110.15, -33.95) -> (102.65, -41.45) construction
  line L3 (102.65, -41.45) -> (110.15, -48.95) construction
  line L4 (113.7209, -45.3791) -> (114.0037, -45.0963)
  line L5 (114.0037, -45.0963) -> (113.1552, -44.2477)
  line L6 (114.0037, -45.0963) -> (114.8523, -45.9448)
  line L7 (114.8523, -45.9448) -> (114.355, -46.4421)
  line L8 (114.355, -46.4421) -> (112.6579, -44.745)
  line L9 (113.1552, -44.2477) -> (112.6579, -44.745)
  line L10 (114.0791, -37.8791) -> (113.7963, -37.5963)
  line L11 (113.7963, -37.5963) -> (112.9477, -38.4448)
  line L12 (113.7963, -37.5963) -> (114.6448, -36.7477)
  line L13 (114.6448, -36.7477) -> (115.2331, -37.336)
  line L14 (115.2331, -37.336) -> (113.536, -39.0331)
  line L15 (112.9477, -38.4448) -> (113.536, -39.0331)
  line L16 (106.5791, -37.5209) -> (106.2963, -37.8037)
  line L17 (106.2963, -37.8037) -> (107.1448, -38.6523)
  line L18 (106.2963, -37.8037) -> (105.4477, -36.9552)
  line L19 (107.1448, -38.6523) -> (107.8727, -37.9243)
  line L20 (107.8727, -37.9243) -> (106.1757, -36.2273)
  line L21 (105.4477, -36.9552) -> (106.1757, -36.2273)
  line L22 (106.2209, -45.0209) -> (106.5037, -45.3037)
  line L23 (106.5037, -45.3037) -> (107.3523, -44.4552)
  line L24 (106.5037, -45.3037) -> (105.6552, -46.1523)
  line L25 (107.3523, -44.4552) -> (106.6403, -43.7432)
  line L26 (106.6403, -43.7432) -> (104.9432, -45.4403)
  line L27 (105.6552, -46.1523) -> (104.9432, -45.4403)
  point P0 (110.15, -48.95)
  point P1 (117.65, -41.45)
  point P2 (110.15, -33.95)
  point P3 (102.65, -41.45)
  dimension "d166" = 0.4
  dimension "d167" = 1.2
  dimension "d168" = 1.2
  dimension "d169" = 0.4
  dimension "d170" = 1.2
  dimension "d171" = 1.2
  dimension "d172" = 0.4
  dimension "d173" = 1.2
  dimension "d174" = 1.2
  dimension "d175" = 0.4
  dimension "d176" = 1.2
  dimension "d177" = 1.2
  constraint coincident P0 L0.start
  constraint coincident P1 L0.end
  constraint coincident P2 L1.end
  constraint coincident P3 L2.end
  constraint coincident L0 L4.start
  constraint parallel L0 L4
  constraint perpendicular L0 L5
  constraint perpendicular L0 L6
  constraint perpendicular L6 L7
  constraint perpendicular L0 L8
  constraint perpendicular L8 L9
  constraint coincident L1 L10.start
  constraint parallel L1 L10
  constraint perpendicular L10 L11
  constraint perpendicular L10 L12
  constraint perpendicular L12 L13
  constraint perpendicular L13 L14
  constraint perpendicular L14 L15
  constraint coincident L2 L16.start
  constraint parallel L2 L16
  constraint perpendicular L2 L17
  constraint perpendicular L2 L18
  constraint perpendicular L17 L19
  constraint perpendicular L19 L20
  constraint perpendicular L20 L21
  constraint coincident L3 L22.start
  constraint parallel L3 L22
  constraint perpendicular L22 L23
  constraint perpendicular L22 L24
  constraint perpendicular L23 L25
  constraint perpendicular L3 L26
  constraint perpendicular L26 L27
  measures "d166" distance of L4.start L4.end
  measures "d167" distance of L4.end L5.end
  measures "d168" distance of L4.end L6.end
  measures "d169" distance of L10.start L10.end
  measures "d170" distance of L10.end L11.end
  measures "d171" distance of L10.end L12.end
  measures "d172" distance of L16.start L16.end
  measures "d173" distance of L16.end L17.end
  measures "d174" distance of L16.end L18.end
  measures "d175" distance of L22.start L22.end
  measures "d176" distance of L22.end L23.end
  measures "d177" distance of L22.end L24.end
extrude "Extrude19" cut sketch "Sketch27" against normal blind 0.5 bodies 4
sketch "Sketch28" plane through (0, 0, 14.6) normal (0, 0, -1) x (1, 0, 0)
  circle A0 centre (117.6453, -56.4453) radius 2.85
  circle A1 centre (102.6547, -56.4453) radius 2.85
  point P0 (117.6453, -56.4453)
  point P1 (102.6547, -56.4453)
  dimension "d180" = 5.7
  dimension "d181" = 5.7
  constraint coincident P0 A0.centre
  constraint coincident P1 A1.centre
  measures "d180" diameter of A0
  measures "d181" diameter of A1
extrude "Extrude20" cut sketch "Sketch28" against normal blind 0.5 bodies 4
sketch "Sketch29" plane through (0, 0, 14.6) normal (0, 0, -1) x (1, 0, 0)
  arc A0 (106.9671, -44.0701) -> (105.2701, -45.7671) centre (102.65, -41.45) ccw
  line L0 (102.65, -41.45) -> (97.6001, -41.4842) construction
  line L1 (97.6001, -41.4842) -> (98.1001, -41.4809)
  line L2 (98.1001, -41.4809) -> (98.115, -43.6717)
  line L3 (98.115, -43.6717) -> (98.1001, -41.4809)
  line L4 (98.1001, -41.4809) -> (98.115, -43.6717)
  line L5 (98.1001, -41.4809) -> (98.115, -43.6717)
  line L6 (97.4084, -39.2946) -> (97.4381, -43.6763)
  line L7 (98.1001, -41.4809) -> (98.0852, -39.29)
  line L8 (98.0852, -39.29) -> (97.4084, -39.2946)
  line L9 (98.115, -43.6717) -> (97.4381, -43.6763)
  line L10 (102.65, -41.45) -> (102.6632, -43.3925) construction
  line L11 (107.1999, -41.4191) -> (107.2148, -43.61)
  line L12 (107.2148, -43.61) -> (107.8916, -43.6054)
  line L13 (107.8619, -39.2237) -> (107.8916, -43.6054)
  line L14 (107.185, -39.2283) -> (107.8619, -39.2237)
  line L15 (107.1999, -41.4191) -> (107.185, -39.2283)
  line L16 (110.15, -33.95) -> (110.15, -40)
  arc A1 (107.5299, -38.2671) -> (105.8329, -36.5701) centre (110.15, -33.95) ccw
  line L17 (110.15, -33.95) -> (110.15, -39)
  line L18 (110.15, -39) -> (110.15, -38.5)
  line L19 (110.15, -38.5) -> (107.6, -38.5)
  line L20 (107.6, -38.5) -> (107.6, -39.1)
  line L21 (107.6, -39.1) -> (112.8, -39.1)
  line L22 (110.15, -38.5) -> (112.8, -38.5)
  line L23 (112.8, -39.1) -> (112.8, -38.5)
  line L24 (110.15, -33.95) -> (108, -33.95) construction
  line L25 (110.15, -33.95) -> (108, -33.95) construction
  line L26 (107.6, -28.8) -> (112.8, -28.8)
  line L27 (112.8, -28.8) -> (112.8, -29.4)
  line L28 (110.15, -29.4) -> (112.8, -29.4)
  line L29 (110.15, -29.4) -> (107.6, -29.4)
  line L30 (107.6, -29.4) -> (107.6, -28.8)
  line L31 (110.15, -48.95) -> (110.15, -54.6)
  line L32 (110.15, -54) -> (110.15, -53.5)
  line L33 (110.15, -53.5) -> (107.9591, -53.5)
  line L34 (110.15, -53.5) -> (112.3364, -53.5)
  line L35 (107.9591, -54.8637) -> (112.3364, -54.8637)
  line L36 (112.3364, -53.5) -> (112.3364, -54.8637)
  line L37 (107.9591, -53.5) -> (107.9591, -54.8637)
  line L38 (110.15, -48.95) -> (110.15, -42.9)
  line L39 (110.15, -43.9) -> (110.15, -44.4)
  line L40 (110.15, -44.4) -> (107.9591, -44.4)
  line L41 (107.9591, -43.8) -> (112.3409, -43.8)
  line L42 (110.15, -44.4) -> (112.3409, -44.4)
  line L43 (112.3409, -44.4) -> (112.3409, -43.8)
  line L44 (107.9591, -44.4) -> (107.9591, -43.8)
  line L45 (117.65, -41.45) -> (111.2969, -41.45)
  line L46 (112.6, -41.45) -> (113.1, -41.45)
  line L47 (113.1, -41.45) -> (113.1, -39)
  line L48 (113.1, -39) -> (112.4, -39)
  line L49 (113.1, -41.45) -> (113.1, -44.1)
  line L50 (113.1, -44.1) -> (112.2, -44.1)
  line L51 (112.2, -44.1) -> (112.2, -39)
  line L52 (112.2, -39) -> (112.4, -39)
  line L53 (117.65, -41.45) -> (124.2, -41.45)
  line L54 (122.7, -41.45) -> (122.2, -41.45)
  line L55 (122.2, -41.45) -> (122.2, -38.1)
  line L56 (122.2, -38.1) -> (123.2, -38.1)
  line L57 (123.2, -38.1) -> (123.2, -45.8)
  line L58 (123.2, -45.8) -> (122.2, -45.8)
  line L59 (122.2, -45.8) -> (122.2, -41.45)
  circle A2 centre (117.65, -41.45) radius 5.05
  circle A3 centre (110.15, -48.95) radius 5.05
  circle A4 centre (102.65, -41.45) radius 5.05
  circle A5 centre (110.15, -33.95) radius 5.05
  point P0 (102.65, -41.45)
  point P1 (110.15, -33.95)
  point P2 (110.15, -48.95)
  point P3 (117.65, -41.45)
  dimension "d184" = 0.5
  dimension "d185" = 0.5
  dimension "d186" = 0.5
  dimension "d187" = 0.5
  dimension "d188" = 0.5
  dimension "d189" = 0.5
  constraint coincident P0 A0.centre
  constraint coincident A0 L0.end
  constraint parallel L0 L1
  constraint perpendicular L1 L2
  constraint parallel L2 L3
  constraint perpendicular L0 L4
  constraint parallel L4 L5
  constraint coincident A0 L7.end
  constraint perpendicular L6 L8
  constraint coincident A0 L2.end
  constraint perpendicular L6 L9
  constraint perpendicular L0 L10
  constraint symmetric L1.end L10 L11.start
  constraint symmetric L7.end L10 L14.start
  constraint symmetric L6.start L10 L13.start
  constraint symmetric L2.end L10 L11.end
  constraint symmetric L6.end L10 L12.end
  constraint coincident P1 L16.start
  constraint coincident L16 L17.end
  constraint coincident A1 L17.end
  constraint parallel L17 L18
  constraint perpendicular L18 L19
  constraint perpendicular L19 L20
  constraint perpendicular L20 L21
  constraint perpendicular L21 L23
  constraint perpendicular L22 L23
  constraint perpendicular L16 L24
  constraint symmetric L18.end L24 L28.start
  constraint symmetric L19.end L24 L29.end
  constraint symmetric L20.end L24 L26.start
  constraint symmetric L21.end L24 L26.end
  constraint symmetric L22.end L24 L27.end
  constraint symmetric P1 L24 L16.start
  constraint symmetric L25.end L24 L24.end
  constraint coincident P2 L31.start
  constraint vertical L31
  constraint coincident L31 L32.start
  constraint parallel L31 L32
  constraint perpendicular L32 L33
  constraint perpendicular L32 L34
  constraint perpendicular L35 L36
  constraint perpendicular L35 L37
  constraint vertical L38
  constraint coincident L38 L39.start
  constraint parallel L38 L39
  constraint perpendicular L38 L40
  constraint perpendicular L41 L43
  constraint perpendicular L41 L44
  constraint coincident P3 L45.start
  constraint horizontal L45
  constraint coincident L45 L46.start
  constraint parallel L45 L46
  constraint perpendicular L46 L47
  constraint perpendicular L47 L48
  constraint perpendicular L46 L49
  constraint perpendicular L49 L50
  constraint perpendicular L21 L51
  constraint perpendicular L51 L52
  constraint horizontal L53
  constraint coincident L53 L54.start
  constraint parallel L53 L54
  constraint perpendicular L53 L55
  constraint perpendicular L55 L56
  constraint perpendicular L53 L57
  constraint perpendicular L57 L58
  constraint perpendicular L53 L59
  constraint coincident L54.start A2
  constraint coincident L32.start A3
  constraint concentric A0 A4
  constraint coincident L0.end A4
  constraint coincident L17.end A5
  measures "d184" distance of L0.end L1.end
  measures "d185" distance of L17.end L18.end
  measures "d186" distance of L32.start L32.end
  measures "d187" distance of L39.start L39.end
  measures "d188" distance of L46.start L46.end
  measures "d189" distance of L54.start L54.end
extrude "Extrude21" add sketch "Sketch29" against normal blind 0.5 contours A0 L11 L15 A4 | A0 L1 L2 L3 L4 L5 A4 | A0 L1 L7 A4 | L16 A1 L17 L18 L22 A5 | L16 A1 L17 L18 L19 A5 | A1 L28 L29 A5 | L45 L46 L47 A2 | L45 L46 L49 A2 | L53 L54 L55 A2 | L53 L54 L59 A2 | L38 L39 L42 A3 | L38 L39 L40 A3 | L31 L32 L33 A3 | L31 L32 L34 A3 bodies 4
sketch "little" plane through (0, 0, 15.5) normal (0, 0, 1) x (-1, 0, 0)
  arc A0 (-31.2, 9.5) -> (-28.2, 12.5) centre (-31.2, 12.5) ccw
  line L0 (-28.2, 12.5) -> (-28.2, 25.9)
  arc A1 (-28.2, 25.9) -> (-31.2, 28.9) centre (-31.2, 25.9) ccw
  line L1 (-31.2, 28.9) -> (-62.7, 28.9)
  arc A2 (-62.7, 28.9) -> (-65.7, 25.9) centre (-62.7, 25.9) ccw
  line L2 (-65.7, 25.9) -> (-65.7, 12.5)
  arc A3 (-65.7, 12.5) -> (-62.7, 9.5) centre (-62.7, 12.5) ccw
  line L3 (-62.7, 9.5) -> (-31.2, 9.5)
  line L4 (-27.2, 4.5) -> (-66.7, 4.5)
  line L5 (-66.7, 4.5) -> (-66.7, 33.9)
  line L6 (-66.7, 33.9) -> (-27.2, 33.9)
  line L7 (-27.2, 33.9) -> (-27.2, 4.5)
  point P0 (-27.2, 4.5)
  point P1 (-66.7, 33.9)
  constraint horizontal L4
  constraint vertical L5
  constraint horizontal L6
  constraint vertical L7
  constraint coincident P1 L5.end
  constraint coincident P0 L4.start
extrude "Extrude22" add sketch "Controls" against normal blind 1 separate body contours L0 L1 L3 L4 L5 L7 L8 L11 L12 L30 L31 L32 L33 A17 A18 makes body 7